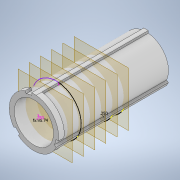
# Autodesk Inventor part: Maze
Saved by Autodesk Inventor 2021 (Build 250183000, 183)
## iProperties
Created: 2020-07-17
Part Number: Maze
Material: Generic
Document SubType Name: Modeling
Designer: saipr
Density: 1 g/cm^3
Appearance: Default
Author: saipr
Autodesk Inventor part; units mm, degrees
ref_plane "YZ Plane" through (0, 0, 0) normal (1, 0, 0) x (0, 1, 0)
ref_plane "XZ Plane" through (0, 0, 0) normal (0, 1, 0) x (-1, 0, 0)
ref_plane "XY Plane" through (0, 0, 0) normal (0, 0, 1) x (1, 0, 0)
sketch "Sketch1" plane through (0, 0, 0) normal (0, 0, 1) x (1, 0, 0)
  circle A0 centre (0, 0) radius 25.4
  circle A1 centre (0, 0) radius 22.225
  line L0 (0, 0) -> (0, 25.4)
  line L1 (0, 0) -> (19.2474, -11.1125)
  line L2 (0, 0) -> (-19.2474, -11.1125)
  line L3 (-19.2474, -11.1125) -> (-21.997, -12.7)
  line L4 (19.2474, -11.1125) -> (21.997, -12.7)
  arc A2 (9.6237, 23.5063) -> (-9.6237, 23.5063) centre (0, 0) ccw
  arc A3 (2.54, 25.2727) -> (-2.54, 25.2727) centre (0, 0) ccw
  line L5 (-2.54, 25.2727) -> (-2.54, 27.8127)
  line L6 (2.54, 25.2727) -> (2.54, 27.8127)
  arc A4 (2.54, 27.8127) -> (-2.54, 27.8127) centre (0, 2.54) ccw
  arc A5 (21.2995, -13.8381) -> (22.9699, -10.8419) centre (0, 0) ccw
  arc A6 (20.5909, -14.872) -> (23.1385, -10.477) centre (0, 0) ccw
  line L7 (-23.1568, -10.4366) -> (-25.3565, -11.7066)
  arc A7 (-25.3565, -11.7066) -> (-22.8165, -16.106) centre (-2.1997, -1.27) ccw
  line L8 (-20.6168, -14.836) -> (-22.8165, -16.106)
  line L9 (20.6168, -14.836) -> (22.8165, -16.106)
  arc A8 (22.8165, -16.106) -> (25.3565, -11.7066) centre (2.1997, -1.27) ccw
  line L10 (23.1568, -10.4366) -> (25.3565, -11.7066)
  point P0 (-2.54, 25.2727)
  point P1 (2.54, 25.2727)
  dimension "d0" = 50.8
  dimension "d1" = 44.45
  dimension "d2" = 120
  dimension "d3" = 120
  dimension "d4" = 2.54
  dimension "d5" = 25.4
  dimension "d6" = 25.4
  dimension "d7" = 5.08
  dimension "d8" = 2.54
  dimension "d9" = 2.54
  dimension "d22" = 360
  constraints: 23 point on circle, 22 end point, 8 centre point, 3 vertical, 2 coincident, 2 collinear, 1 concentric, 35 other
  measures "d1" diameter of A1
  measures "d2" angle of L1 L0
  measures "d3" angle of L0 L2
  measures "d4" distance of L5.start L5.end
  measures "d5" radius of A2
  measures "d6" radius of A4
  measures "d7" distance between parallel lines of L6 L5
  measures "d8" distance of L6.start L6.end
  measures "d9" distance between parallel lines of L6 L0
extrude "Extrusion1" add sketch "Sketch1" along normal blind 127 contours A0 L4 A1 L0 | L10 A8 L9 A0 | A0 L5 A4 L6 | L0 A1 L3 A0 | A0 L3 A1 L4 | A0 L8 A7 L7
sketch "Sketch2" plane through (0, 0, 127) normal (0, 0, 1) x (1, 0, 0)
  line L0 (-2.54, 27.8127) -> (-2.54, 25.2727) projected
  line L1 (-23.1568, -10.4366) -> (-25.3565, -11.7066) projected
  arc A0 (-2.54, 25.2727) -> (-23.1568, -10.4366) centre (0, 0) ccw
  arc A1 (-2.54, 25.2727) -> (-23.1568, -10.4366) centre (0, 0) ccw projected
  line L2 (25.3565, -11.7066) -> (23.1568, -10.4366) projected
  line L3 (2.54, 25.2727) -> (2.54, 27.8127) projected
  arc A2 (23.1568, -10.4366) -> (2.54, 25.2727) centre (0, 0) ccw
  arc A3 (-20.6168, -14.836) -> (20.6168, -14.836) centre (0, 0) ccw projected
  arc A4 (-20.6168, -14.836) -> (20.6168, -14.836) centre (0, 0) ccw
  arc A5 (23.1568, -10.4366) -> (2.54, 25.2727) centre (0, 0) ccw projected
  arc A6 (23.1568, -10.4366) -> (25.0218, -4.3667) centre (0, 0) ccw
  arc A7 (25.0218, -4.3667) -> (2.54, 25.2727) centre (0, 0) ccw
  arc A8 (25.3565, -11.7066) -> (2.54, 27.8127) centre (0, 0) ccw
  arc A9 (-20.6168, -14.836) -> (-16.2926, -19.4862) centre (0, 0) ccw
  arc A10 (-25.3565, -11.7066) -> (-22.8165, -16.106) centre (-2.1997, -1.27) ccw projected
  arc A11 (22.8165, -16.106) -> (25.3565, -11.7066) centre (2.1997, -1.27) ccw projected
  arc A12 (-22.8165, -16.106) -> (22.8165, -16.106) centre (0, 0) ccw
  arc A13 (-16.2926, -19.4862) -> (20.6168, -14.836) centre (0, 0) ccw
  arc A14 (-2.54, 25.2727) -> (-8.7292, 23.8529) centre (0, 0) ccw
  arc A15 (-2.54, 27.8127) -> (-25.3565, -11.7066) centre (0, 0) ccw
  arc A16 (-8.7292, 23.8529) -> (-23.1568, -10.4366) centre (0, 0) ccw
  arc A17 (-20.6168, -14.836) -> (20.6168, -14.836) centre (0, 0) ccw projected
  line L4 (-2.54, 25.2727) -> (-5.2844, 24.9969)
  line L5 (-8.7292, 23.8529) -> (-6.0639, 24.8283)
  line L6 (-9.8364, 26.1389) -> (-8.7292, 23.8529)
  line L7 (-2.54, 25.2727) -> (-2.54, 27.8127)
  line L8 (25.0218, -4.3667) -> (24.1203, -9.5324)
  line L9 (25.0218, -4.3667) -> (27.5551, -4.5509)
  line L10 (-16.2926, -19.4862) -> (-20.425, -16.0311)
  line L11 (-16.2926, -19.4862) -> (-17.7188, -21.588)
  line L12 (20.6168, -14.836) -> (22.8165, -16.106)
  line L13 (-20.6168, -14.836) -> (-16.2926, -19.4862)
  point P0 (25.0218, -4.3667)
  point P1 (-8.7292, 23.8529)
  point P2 (-16.2926, -19.4862)
  dimension "d26" = 6.35
  dimension "d27" = 6.35
  dimension "d28" = 6.35
  dimension "d31" = 25.4
  dimension "d32" = 2.54
  dimension "d34" = 95.74
  dimension "d35" = 95.74
  dimension "d36" = 95.74
  constraints: 31 point on circle, 20 end point, 12 centre point, 12 tangent, 6 concentric, 1 collinear
  measures "d26" distance of L2.end L8.start
  measures "d27" distance of L13.start L10.start
  measures "d28" distance of L0.end L5.start
  measures "d31" radius of A1
  measures "d32" distance of L0.start L0.end
  measures "d34" angle of L6 L5
  measures "d35" angle of L9 L8
  measures "d36" angle of L11 L10
extrude "Extrusion2" add sketch "Sketch2" against normal blind 6.35 contours L6 A0 L1 A15 | L9 A2 L3 A8 | A3 L12 A12 L11
ref_plane "Work Plane1" through (0, 0, 114.3) normal (0, 0, 1) x (1, 0, 0)
sketch "Sketch3" plane through (0, 0, 114.3) normal (0, 0, 1) x (1, 0, 0)
  arc A0 (-20.6168, -14.836) -> (20.6168, -14.836) centre (0, 0) ccw
  arc A1 (-25.3565, -11.7066) -> (-22.8165, -16.106) centre (-2.1997, -1.27) ccw projected
  arc A2 (22.8165, -16.106) -> (25.3565, -11.7066) centre (2.1997, -1.27) ccw projected
  arc A3 (-22.8165, -16.106) -> (22.8165, -16.106) centre (0, 0) ccw
  arc A4 (-17.7188, -21.588) -> (22.8165, -16.106) centre (0, 0) ccw projected
  arc A5 (-20.6168, -14.836) -> (20.6168, -14.836) centre (0, 0) ccw projected
  line L0 (20.6168, -14.836) -> (17.8083, -18.7389)
  line L1 (20.6168, -14.836) -> (16.2926, -19.4862)
  line L2 (16.2926, -19.4862) -> (20.2443, -16.1821)
  line L3 (16.2926, -19.4862) -> (17.7188, -21.588)
  line L4 (-20.6168, -14.836) -> (-22.8165, -16.106)
  line L5 (20.6168, -14.836) -> (22.8165, -16.106)
  dimension "d40" = 6.35
  dimension "d41" = 95.74
  constraints: 12 end point, 6 point on circle, 2 centre point, 2 tangent, 1 concentric
  measures "d40" distance of L0.start L1.end
  measures "d41" angle of L3 L2
extrude "Extrusion3" [suppressed]
ref_plane "Work Plane2" through (0, 0, 101.6) normal (0, 0, 1) x (1, 0, 0)
sketch "Sketch4" plane through (0, 0, 101.6) normal (0, 0, 1) x (1, 0, 0)
  line L0 (-22.8165, -16.106) -> (-20.6168, -14.836) projected
  arc A0 (22.8165, -16.106) -> (25.3565, -11.7066) centre (2.1997, -1.27) ccw projected
  arc A1 (-22.8165, -16.106) -> (22.8165, -16.106) centre (0, 0) ccw
  arc A2 (-20.6168, -14.836) -> (-16.2926, -19.4862) centre (0, 0) ccw projected
  line L1 (2.54, 25.2727) -> (2.54, 27.8127) projected
  arc A3 (22.8165, -16.106) -> (2.54, 27.8127) centre (0, 0) ccw
  arc A4 (2.54, 27.8127) -> (-22.8165, -16.106) centre (0, 0) ccw
  line L2 (-22.8165, -16.106) -> (-20.6168, -14.836)
  arc A5 (-20.6168, -14.836) -> (-16.2926, -19.4862) centre (0, 0) ccw
  line L3 (-20.6168, -14.836) -> (-16.2926, -19.4862)
  line L4 (-16.2926, -19.4862) -> (-17.7173, -21.5892)
  line L5 (-16.2926, -19.4862) -> (-19.4492, -16.851)
  arc A6 (-20.6168, -14.836) -> (20.6168, -14.836) centre (0, 0) ccw
  arc A7 (-22.8165, -16.106) -> (22.8165, -16.106) centre (0, 0) ccw
  line L6 (22.8165, -16.106) -> (20.6168, -14.836)
  point P0 (-16.2926, -19.4862)
  point P1 (-16.2926, -19.4862)
  point P2 (-16.2926, -19.4862)
  dimension "d47" = 6.35
  dimension "d48" = 95.74
  constraints: 16 point on circle, 10 end point, 6 centre point, 6 concentric
  measures "d47" distance of L0.end L3.end
  measures "d48" angle of L4 L5
extrude "Extrusion4" [suppressed]
ref_plane "Work Plane3" through (0, 0, 88.9) normal (0, 0, 1) x (1, 0, 0)
sketch "Sketch5" plane through (0, 0, 88.9) normal (0, 0, 1) x (1, 0, 0)
  arc A0 (-25.3565, -11.7066) -> (-22.8165, -16.106) centre (-2.1997, -1.27) ccw projected
  arc A1 (22.8165, -16.106) -> (25.3565, -11.7066) centre (2.1997, -1.27) ccw projected
  arc A2 (-20.6168, -14.836) -> (20.6168, -14.836) centre (0, 0) ccw projected
  arc A3 (-20.6168, -14.836) -> (20.6168, -14.836) centre (0, 0) ccw
  arc A4 (-22.8165, -16.106) -> (22.8165, -16.106) centre (0, 0) ccw
  line L0 (20.6168, -14.836) -> (17.9529, -18.5379)
  line L1 (20.6168, -14.836) -> (16.2926, -19.4862)
  line L2 (16.2926, -19.4862) -> (20.1998, -16.2193)
  line L3 (16.2926, -19.4862) -> (17.7188, -21.588)
  line L4 (-20.6168, -14.836) -> (-22.8165, -16.106)
  point P0 (-22.8165, -16.106)
  dimension "d52" = 6.35
  constraints: 10 end point, 7 point on circle, 2 centre point, 2 tangent, 1 concentric
  measures "d52" distance of L0.start L1.end
extrude "Extrusion5" [suppressed]
ref_plane "Work Plane4" through (0, 0, 76.2) normal (0, 0, 1) x (1, 0, 0)
sketch "Sketch6" plane through (0, 0, 76.2) normal (0, 0, 1) x (1, 0, 0)
  arc A0 (-25.3565, -11.7066) -> (-22.8165, -16.106) centre (-2.1997, -1.27) ccw projected
  arc A1 (-22.8165, -16.106) -> (22.8165, -16.106) centre (0, 0) ccw
  arc A2 (-17.7188, -21.588) -> (22.8165, -16.106) centre (0, 0) ccw projected
  arc A3 (-20.6168, -14.836) -> (20.6168, -14.836) centre (0, 0) ccw projected
  arc A4 (-20.6168, -14.836) -> (20.6168, -14.836) centre (0, 0) ccw
  line L0 (-20.6168, -14.836) -> (-22.8165, -16.106)
  line L1 (22.8165, -16.106) -> (20.6168, -14.836)
  line L2 (-17.7188, -21.588) -> (-16.2926, -19.4862) projected
  line L3 (-17.7188, -21.588) -> (-16.2926, -19.4862)
  constraints: 6 end point, 4 point on circle, 2 centre point, 1 collinear, 1 concentric
extrude "Extrusion6" [suppressed]
ref_plane "Work Plane5" through (0, 0, 63.5) normal (0, 0, 1) x (1, 0, 0)
sketch "Sketch7" plane through (0, 0, 63.5) normal (0, 0, 1) x (1, 0, 0)
  arc A0 (-25.3565, -11.7066) -> (-22.8165, -16.106) centre (-2.1997, -1.27) ccw projected
  arc A1 (22.8165, -16.106) -> (25.3565, -11.7066) centre (2.1997, -1.27) ccw projected
  arc A2 (-22.8165, -16.106) -> (22.8165, -16.106) centre (0, 0) ccw
  arc A3 (-17.7188, -21.588) -> (22.8165, -16.106) centre (0, 0) ccw projected
  line L0 (-22.8165, -16.106) -> (-20.6168, -14.836) projected
  arc A4 (-20.6168, -14.836) -> (20.6168, -14.836) centre (0, 0) ccw projected
  arc A5 (-20.6168, -14.836) -> (20.6168, -14.836) centre (0, 0) ccw
  line L1 (-22.8165, -16.106) -> (-20.6168, -14.836)
  line L2 (22.8165, -16.106) -> (20.6168, -14.836)
  line L3 (20.6168, -14.836) -> (16.2926, -19.4862)
  line L4 (18.1575, -21.2203) -> (16.2926, -19.4862)
  dimension "d60" = 6.35
  constraints: 8 end point, 6 point on circle, 2 centre point, 2 concentric
  measures "d60" distance of L2.end L3.end
ref_plane "Work Plane6" through (0, 0, 50.8) normal (0, 0, 1) x (1, 0, 0)
sketch "Sketch8" plane through (0, 0, 50.8) normal (0, 0, 1) x (1, 0, 0)
  line L0 (-22.8165, -16.106) -> (-20.6168, -14.836) projected
  arc A0 (-20.6168, -14.836) -> (20.6168, -14.836) centre (0, 0) ccw projected
  arc A1 (-20.6168, -14.836) -> (20.6168, -14.836) centre (0, 0) ccw
  arc A2 (-17.7188, -21.588) -> (22.8165, -16.106) centre (0, 0) ccw projected
  arc A3 (-22.8165, -16.106) -> (22.8165, -16.106) centre (0, 0) ccw
  line L1 (-22.8165, -16.106) -> (-20.6168, -14.836)
  line L2 (-16.2926, -19.4862) -> (-17.7188, -21.588) projected
  line L3 (-17.7188, -21.588) -> (-16.2926, -19.4862)
  arc A4 (22.8165, -16.106) -> (25.3565, -11.7066) centre (2.1997, -1.27) ccw projected
  line L4 (20.6168, -14.836) -> (22.8165, -16.106)
  constraints: 6 end point, 4 point on circle, 2 centre point, 2 concentric, 1 collinear
equation "\"d6\" = d5"
equation "\"d8\" = d4"
equation "\"d9\" = 0.5 * d7"
equation "\"d35\" = d34"
equation "\"d36\" = d34"
equation "\"d41\" = d35"
equation "\"d48\" = d36"
body "Solid1"
